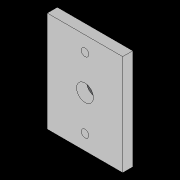
# Autodesk Inventor part: Soporte Pistón
Saved by Autodesk Inventor 2021 (Build 250183000, 183)
## iProperties
Created: 2021-05-02
Part Number: Soporte Pistón
Material: Generic
Document SubType Name: Modeling
Designer: maaro
Density: 1 g/cm^3
Appearance: Default
Author: maaro
Autodesk Inventor part; units mm, degrees
ref_plane "YZ Plane" through (0, 0, 0) normal (1, 0, 0) x (0, 1, 0)
ref_plane "XZ Plane" through (0, 0, 0) normal (0, 1, 0) x (-1, 0, 0)
ref_plane "XY Plane" through (0, 0, 0) normal (0, 0, 1) x (1, 0, 0)
ref_plane "Work Plane1" through (0, 0, 0) normal (0, 0, 1) x (1, 0, 0)
sketch "Sketch1" plane through (0, 0, 0) normal (0, 0, 1) x (1, 0, 0)
  circle A0 centre (0, -16.8) radius 16.8
  circle A1 centre (0, 52.9) radius 8
  line L0 (-75, -117.1) -> (75, -117.1)
  line L1 (75, -117.1) -> (75, 82.9)
  line L2 (75, 82.9) -> (-75, 82.9)
  line L3 (-75, 82.9) -> (-75, -117.1)
  circle A2 centre (0, -87.1) radius 8
  point P0 (0, 0)
extrude "Extrusion1" add sketch "Sketch1" along normal blind 20
body "Solid1"
